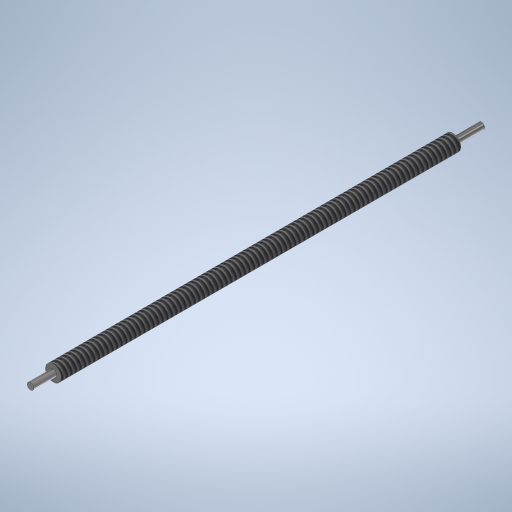
# Autodesk Inventor part: Eixo roscado
Saved by Autodesk Inventor 2023 (Build 270158000, 158)
## iProperties
Created: 2023-03-17
Part Number: Eixo roscado
Material: Aço galvanizado
Document SubType Name: Sheet Metal
Designer: Mateus
Density: 7.85 g/cm^3
Sheet Metal Rule: Default_mm
Appearance: Galvanizado
Mass: 432.933 g
Surface Area: 165.499 cm^2
Volume: 55.1507 cm^3
Author: Mateus
Autodesk Inventor part; units mm, degrees
ref_plane "YZ Plane" through (0, 0, 0) normal (1, 0, 0) x (0, 1, 0)
ref_plane "XZ Plane" through (0, 0, 0) normal (0, 1, 0) x (-1, 0, 0)
ref_plane "XY Plane" through (0, 0, 0) normal (0, 0, 1) x (1, 0, 0)
sketch "Esboço1" plane through (0, 0, 0) normal (0, 1, 0) x (-1, 0, 0)
  line L0 (0, 0) -> (3, 0)
  line L1 (3, 0) -> (3, -20)
  line L2 (3, -20) -> (7, -20)
  line L3 (7, -20) -> (7, -370)
  line L4 (7, -370) -> (3, -370)
  line L5 (3, -370) -> (3, -395)
  line L6 (3, -395) -> (0, -395)
  line L7 (0, -395) -> (0, 0)
  dimension "d0" = 3
  dimension "d1" = 20
  dimension "d2" = 4
  dimension "d3" = 350
  dimension "d4" = 4
  dimension "d5" = 25
  constraints: 16 end point, 6 perpendicular, 2 horizontal
  measures "d0" distance of L0.start L0.end
  measures "d1" distance of L0.end L1.end
  measures "d2" distance of L1.end L2.end
  measures "d3" distance of L2.end L3.end
  measures "d4" distance of L3.end L4.end
  measures "d5" distance of L4.end L5.end
revolve "Revolução1" add sketch "Esboço1" angle 360 about axis through (0, 0, -395) along (0, 0, 1)
sketch "Sketch3" plane through (0, 0, 0) normal (1, 0, 0) x (0, 1, 0)
  line L0 (-7, -20) -> (7, -20) projected
  arc A0 (6.5, -20.866) -> (6.5, -22.5981) centre (7, -21.7321) ccw
  line L1 (7, -20) -> (7, -370) projected
  arc A1 (6.5, -20.866) -> (7, -20) centre (6, -20) ccw
  arc A2 (7, -23.4641) -> (6.5, -22.5981) centre (6, -23.4641) ccw
  line L2 (-7, -20) -> (-7, -370) projected
  point P0 (0, 0)
  dimension "d10" = 2
  dimension "d11" = 1
  dimension "d12" = 1
  dimension "d13" = 0
  constraints: 6 point on circle, 4 equal radius, 3 centre point, 3 point on line
  measures "d10" diameter of A0
  measures "d11" horizontal distance of A1.centre A0.centre
  measures "d12" horizontal distance of A0.centre A2.centre
  measures "d13" distance from line of L0 A1.centre
coil "Coil1" [suppressed]
thread "Thread2" size "M52x4" class "6g" standard "ISO Metric profile" full length
equation "\"d11\" = 0.5 * d10"
equation "\"d12\" = d11"
equation "\"Raio_vergadura\" = Espessura"
equation "\"Largura_alívio_de_vergadura\" = Espessura"
equation "\"Profundidade_alívio_de_vergadura\" = 0.5 * Espessura"
equation "\"Tamanho_alívio_de_dobra\" = 4 * Espessura"
equation "\"Remanescente_mínimo\" = 2 * Espessura"
equation "\"Raiodetransição\" = Raio_vergadura"
equation "\"Tamanho_de_raio_de_Jacobi\" = Raio_vergadura"
equation "\"TamanhoFolga\" = Espessura"
equation "\"Espessura\" = 0.5"
